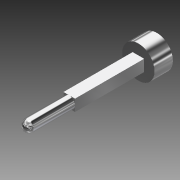
# Autodesk Inventor part: boltV5
Saved by Autodesk Inventor 2013 (Build 170138000, 138)
## iProperties
Created: 2013-05-01
Part Number: boltV5
Material: Nickel-Copper Alloy 400
Document SubType Name: Modeling
Designer: 120pa
Density: 1 g/cm^3
Author: 120pa
Autodesk Inventor part; units mm, degrees
ref_plane "YZ Plane" through (0, 0, 0) normal (1, 0, 0) x (0, 1, 0)
ref_plane "XZ Plane" through (0, 0, 0) normal (0, 1, 0) x (-1, 0, 0)
ref_plane "XY Plane" through (0, 0, 0) normal (0, 0, 1) x (1, 0, 0)
sketch "Sketch2" plane through (0, 0, 0) normal (0, 1, 0) x (-1, 0, 0)
  line L0 (8.0742, -13.0068) -> (8.0742, 15.9932)
  line L1 (9.3242, 14.7432) -> (9.3242, -9.0068)
  line L2 (9.3242, -9.0068) -> (11.5742, -9.0068)
  line L3 (11.5742, -9.0068) -> (11.5742, -13.0068)
  line L4 (11.5742, -13.0068) -> (8.0742, -13.0068)
  arc A0 (9.3242, 14.7432) -> (8.0742, 15.9932) centre (8.0742, 14.7432) ccw
  point P0 (0, 0)
  dimension "d13" = 29
  dimension "d15" = 1.25
  dimension "d16" = 3.5
  dimension "d17" = 4
  constraints: 10 end point, 4 perpendicular, 2 point on circle, 1 centre point, 1 point on line, 1 tangent
  measures "d13" distance of L0.start L0.end
  measures "d15" distance between parallel lines of L1 L0
  measures "d16" distance of L3.end L0.start
  measures "d17" distance of L2.end L3.end
revolve "Revolution2" add sketch "Sketch2" angle 360 about axis through (-8.0742, 0, -13.0068) along (0, 0, 1)
sketch "Sketch3" plane through (-8.0742, 0, -9.0068) normal (0, 0, 1) x (1, 0, 0)
  circle A0 centre (0, 0) radius 1.25 projected
  line L0 (-1.25, 1.25) -> (1.25, 1.25)
  line L1 (1.25, 1.25) -> (1.25, -1.25)
  line L2 (1.25, -1.25) -> (-1.25, -1.25)
  line L3 (-1.25, -1.25) -> (-1.25, 1.25)
  circle A1 centre (0, 0) radius 1.25 projected
  point P0 (8.0742, 0)
  constraints: 8 end point, 4 tangent, 3 perpendicular
extrude "Extrusion1" add sketch "Sketch3" along normal blind 15 contours L1 L2 A0 | A0 L0 L1 | A0 L3 L0 | L2 L3 A0
body "Solid2"
